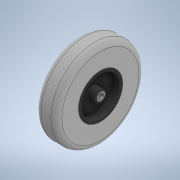
# Autodesk Inventor part: wheel
Saved by Autodesk Inventor 2022 (Build 260153000, 153)
## iProperties
Created: 2021-12-05
Part Number: wheel
Material: Generic
Document SubType Name: Modeling
Designer: Vedic
Density: 1 g/cm^3
Appearance: Default
Author: Vedic
Autodesk Inventor part; units mm, degrees
ref_plane "YZ Plane" through (0, 0, 0) normal (1, 0, 0) x (0, 1, 0)
ref_plane "XZ Plane" through (0, 0, 0) normal (0, 1, 0) x (-1, 0, 0)
ref_plane "XY Plane" through (0, 0, 0) normal (0, 0, 1) x (1, 0, 0)
sketch "Sketch3" plane through (0, 0, 0) normal (1, 0, 0) x (0, 1, 0)
  circle A0 centre (0, 0) radius 12.7
  circle A1 centre (0, 0) radius 50.8
  circle A2 centre (0, 0) radius 101.6
  circle A3 centre (0, 0) radius 44.45
  circle A4 centre (0, 0) radius 9.525
  circle A5 centre (0, 0) radius 6.35
  dimension "d10" = 25.4
  dimension "d11" = 101.6
  dimension "d12" = 203.2
  dimension "d13" = 88.9
  dimension "d14" = 19.05
  dimension "d15" = 12.7
  constraints: 6 centre point, 6 coincident
  measures "d10" diameter of A0
  measures "d11" diameter of A1
  measures "d12" diameter of A2
  measures "d13" diameter of A3
  measures "d14" diameter of A4
  measures "d15" diameter of A5
extrude "Extrusion4" add sketch "Sketch3" along normal mid plane 49.53 contours A0 | A1
extrude "Extrusion5" add sketch "Sketch3" along normal mid plane 12.7 contours A3
extrude "Extrusion6" add sketch "Sketch3" along normal mid plane 48.26 contours A2
extrude "Extrusion7" add sketch "Sketch3" along normal mid plane 50.8 contours A4
fillet "Fillet1" radius 12.7 2 edges at (24.13, -101.6, 0) (-24.13, -101.6, 0)
body "Solid2"
